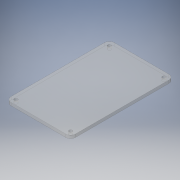
# Autodesk Inventor part: LCD_Cover
Saved by Autodesk Inventor 2016 (Build 200138000, 138)
## iProperties
Created: 2016-04-09
Part Number: LCD_Cover
Material: Polycarbonate, Clear
Document SubType Name: Modeling
Designer: agmle
Density: 1.2 g/cm^3
Appearance: Polycarbonate - Clear
Mass: 24.1373 g
Surface Area: 145.214 cm^2
Volume: 20.1144 cm^3
LCD_Cover_Thickness: 0.118 in
LCD_Cover_Hole_Diameter: 0.129 in
LCD_PCB_Vertical_Hole_Spacing: 2.165 in
LCD_PCB_Horizontal_Hole_Spacing: 3.701 in
Author: agmle
Autodesk Inventor part; units mm, degrees
ref_plane "YZ Plane" through (0, 0, 0) normal (1, 0, 0) x (0, 1, 0)
ref_plane "XZ Plane" through (0, 0, 0) normal (0, 1, 0) x (-1, 0, 0)
ref_plane "Work Plane2" through (-36.5132, 1.6, 47.4786) normal (0, 1, 0) x (1, 0, 0)
sketch "Sketch1" plane through (-36.5132, 1.6, 47.4786) normal (0, 1, 0) x (1, 0, 0)
  line L0 (-22.6989, -29.8949) -> (32.3011, -29.8949)
  line L1 (37.3011, -24.8949) -> (37.3011, 69.1051)
  line L2 (32.3011, 74.1051) -> (-22.6989, 74.1051)
  line L3 (-27.6989, 69.1051) -> (-27.6989, -24.8949)
  arc A0 (-27.6989, -24.8949) -> (-22.6989, -29.8949) centre (-22.6989, -24.8949) ccw
  arc A1 (-22.6989, 74.1051) -> (-27.6989, 69.1051) centre (-22.6989, 69.1051) ccw
  arc A2 (37.3011, 69.1051) -> (32.3011, 74.1051) centre (32.3011, 69.1051) ccw
  arc A3 (32.3011, -29.8949) -> (37.3011, -24.8949) centre (32.3011, -24.8949) ccw
  line L4 (-22.6989, -24.8949) -> (32.3011, -24.8949) construction
  line L5 (32.3011, -24.8949) -> (32.3011, 69.1051) construction
  line L6 (32.3011, 69.1051) -> (-22.6989, 69.1051) construction
  line L7 (-22.6989, 69.1051) -> (-22.6989, -24.8949) construction
  dimension "d2" = 5
  dimension "d5" = 94
  dimension "d6" = 55
  constraints: 16 end point, 8 point on circle, 8 tangent, 4 centre point, 4 parallel, 3 equal radius, 2 perpendicular, 1 horizontal
  measures "d2" radius of A0
  measures "d5" distance of L6.end L4.start
  measures "d6" distance of L4.start L4.end
extrude "Extrusion1" add sketch "Sketch1" along normal blind 3
sketch "Sketch2" plane through (-36.5132, 1.6, 47.4786) normal (0, -1, 0) x (1, 0, 0)
  arc A0 (-22.6989, 29.8949) -> (-27.6989, 24.8949) centre (-22.6989, 24.8949) ccw construction
  arc A1 (-27.6989, -69.1051) -> (-22.6989, -74.1051) centre (-22.6989, -69.1051) ccw construction
  arc A2 (32.3011, -74.1051) -> (37.3011, -69.1051) centre (32.3011, -69.1051) ccw construction
  arc A3 (37.3011, 24.8949) -> (32.3011, 29.8949) centre (32.3011, 24.8949) ccw construction
  constraints: 4 coincident
hole "Hole1" at (-59.2121, 1.6, -21.6265) at (-4.2121, 1.6, 72.3735) at (-59.2121, 1.6, 72.3735) at (-4.2121, 1.6, -21.6265) direction (0, 1, 0) diameter 3.2766 end through all clearance for "Socket Head Cap Screw" size "#4" standard "Ansi Unified Screw Threads"
equation "\"d5\" = LCD_PCB_Horizontal_Hole_Spacing"
equation "\"d6\" = LCD_PCB_Vertical_Hole_Spacing"
equation "\"LCD_PCB_Horizontal_Hole_Spacing\" = 94"
equation "\"LCD_PCB_Vertical_Hole_Spacing\" = 55"
body "Solid1"
